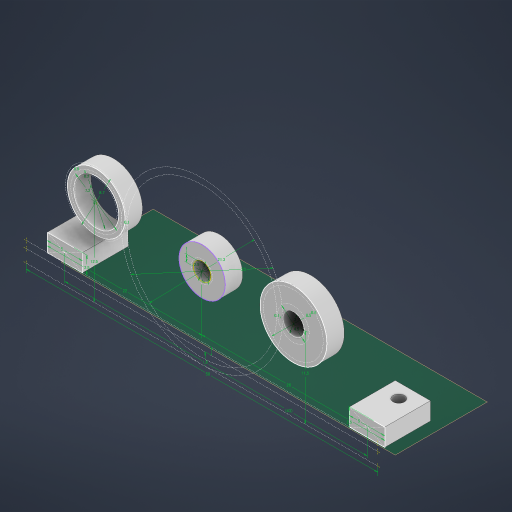
# Autodesk Inventor part: motormount
Saved by Autodesk Inventor 2023.5 (Build 275446000, 446)
## iProperties
Created: 2025-01-19
Part Number: motormount
Material: 一般
Document SubType Name: Modeling
Designer: IshiiLabHonda
Density: 1 g/cm^3
Appearance: 既定
Author: IshiiLabHonda
Autodesk Inventor part; units mm, degrees
ref_plane "YZ Plane" through (0, 0, 0) normal (1, 0, 0) x (0, 1, 0)
ref_plane "XZ Plane" through (0, 0, 0) normal (0, 1, 0) x (-1, 0, 0)
ref_plane "XY Plane" through (0, 0, 0) normal (0, 0, 1) x (1, 0, 0)
sketch "スケッチ1" plane through (0, 0, 0) normal (0, 0, 1) x (1, 0, 0)
  circle A0 centre (0, 0) radius 10.65 construction
  line L0 (0, 0) -> (0, 1) construction
  line L1 (0, 0) -> (1, 0) construction
  circle A1 centre (13, 0) radius 2.25 construction
  circle A2 centre (-15.0669, 1) radius 4.35 construction
  circle A3 centre (0, 0) radius 11.5 construction
  line L2 (-25, -11.5) -> (25, -11.5) construction
  line L3 (-25, -9.7) -> (25, -9.7) construction
  line L4 (-25, -8.7) -> (25, -8.7) construction
  dimension "d0" = 1
  dimension "d2" = 1
  dimension "d3" = 21.3
  dimension "d5" = 4.5
  dimension "d6" = 0.1
  dimension "d7" = 8.7
  dimension "d8" = 0.1
  dimension "d9" = 23
  dimension "d10" = 50
  dimension "d11" = 1.8
  dimension "d12" = 1
  dimension "d46" = 12.5
  dimension "d47" = 11.5
  constraints: 10 end point, 5 parallel, 4 centre point, 4 coincident, 3 symmetric about line, 1 perpendicular, 1 tangent, 1 vertical
  measures "d0" distance of L0.start L0.end
  measures "d2" distance of L0.start L1.end
  measures "d3" diameter of A0
  measures "d5" diameter of A1
  measures "d7" diameter of A2
  measures "d9" diameter of A3
  measures "d10" distance of L2.start L2.end
  measures "d11" distance between parallel lines of L2 L3
  measures "d12" distance between parallel lines of L3 L4
  measures "d46" distance from line of L2 A2.centre
  measures "d47" distance from line of L2 A1.centre
sketch "スケッチ2" plane through (0, 0, 0) normal (0, 0, 1) x (1, 0, 0)
  circle A0 centre (-15.0669, 1) radius 4.35 construction
  line L0 (0, 0) -> (0, 1) construction
  circle A1 centre (0, 0) radius 10.65 construction
  circle A2 centre (0, 0) radius 11.5 construction
  line L1 (-25, -8.7) -> (25, -8.7) construction
  line L2 (-25, -9.7) -> (25, -9.7) construction
  line L3 (-25, -11.5) -> (25, -11.5) construction
  line L4 (0, 0) -> (1, 0) construction
  circle A3 centre (13, 0) radius 2.25 construction
  circle A4 centre (13, 0) radius 4.25 construction
  circle A5 centre (-15.0669, 1) radius 3.6 construction
  circle A6 centre (-15.0669, 1) radius 3 construction
  circle A7 centre (0, 0) radius 1.25 construction
  circle A8 centre (0, 0) radius 1.5 construction
  dimension "d13" = 8.5
  dimension "d14" = 7.2
  dimension "d15" = 6
  dimension "d27" = 2.5
  dimension "d28" = 3
  constraints: 5 centre point, 5 coincident
  measures "d13" diameter of A4
  measures "d14" diameter of A5
  measures "d15" diameter of A6
  measures "d27" diameter of A7
  measures "d28" diameter of A8
sketch "スケッチ3" plane through (0, 0, 0) normal (0, 0, 1) x (1, 0, 0)
  circle A0 centre (-15.0669, 1) radius 4.35 construction
  line L0 (0, 0) -> (0, 1) construction
  line L1 (0, 0) -> (1, 0) construction
  line L2 (-25, -11.5) -> (25, -11.5) construction
  line L3 (-25, -9.7) -> (25, -9.7) construction
  line L4 (-25, -8.7) -> (25, -8.7) construction
  circle A1 centre (13, 0) radius 2.25 construction
  circle A2 centre (0, 0) radius 10.65 construction
  circle A3 centre (0, 0) radius 11.5 construction
  circle A4 centre (-15.0669, 1) radius 4.35 construction
  line L5 (0, 0) -> (0, 1) construction
  circle A5 centre (0, 0) radius 10.65 construction
  circle A6 centre (0, 0) radius 11.5 construction
  line L6 (-25, -8.7) -> (25, -8.7) construction
  line L7 (-25, -9.7) -> (25, -9.7) construction
  line L8 (-25, -11.5) -> (25, -11.5) construction
  line L9 (0, 0) -> (1, 0) construction
  circle A7 centre (13, 0) radius 2.25 construction
  circle A8 centre (13, 0) radius 4.25 construction
  circle A9 centre (-15.0669, 1) radius 3.6 construction
  circle A10 centre (-15.0669, 1) radius 3 construction
  line L10 (-22, -6.2) -> (-17, -6.2)
  line L11 (-17, -6.2) -> (-17, -8.7)
  line L12 (-22, -8.7) -> (-22, -6.2)
  line L13 (21, -6.2) -> (26, -6.2)
  line L14 (26, -6.2) -> (26, -8.7)
  line L15 (21, -8.7) -> (21, -6.2)
  line L16 (-22, -6.2) -> (-17, -8.7) construction
  line L17 (-22, -8.7) -> (-17, -6.2) construction
  line L18 (21, -6.2) -> (26, -8.7) construction
  line L19 (21, -8.7) -> (26, -6.2) construction
  line L20 (-22, -8.7) -> (-17, -8.7)
  line L21 (21, -8.7) -> (26, -8.7)
  circle A11 centre (-15.0669, 1) radius 3.2
  circle A12 centre (-15.0669, 1) radius 4.1
  circle A13 centre (13, 0) radius 4.75
  circle A14 centre (0, 0) radius 3.2895
  circle A15 centre (0, 0) radius 1.25 projected
  circle A16 centre (13, 0) radius 1.5
  point P0 (-19.5, -7.45)
  point P1 (23.5, -7.45)
  point P2 (15.3415, -6)
  point P3 (15, -6.1912)
  dimension "d17" = 5
  dimension "d18" = 5
  dimension "d19" = 2.5
  dimension "d20" = 2.5
  dimension "d22" = 22
  dimension "d23" = 26
  dimension "d24" = 0.2
  dimension "d25" = 0.5
  dimension "d26" = 0.5
  dimension "d31" = 3
  dimension "d39" = 43
  constraints: 24 end point, 5 centre point, 5 coincident, 4 point on line, 3 parallel, 2 midpoint, 2 perpendicular, 4 other
  measures "d17" distance between parallel lines of L11 L12
  measures "d18" distance between parallel lines of L15 L14
  measures "d19" distance between parallel lines of L6 L10
  measures "d20" distance between parallel lines of L4 L13
  measures "d22" distance of the line from the sketch origin of L12
  measures "d23" distance of the line from the sketch origin of L14
  measures "d24" radial gap between concentric circles of A10 A11
  measures "d25" radial gap between concentric circles of A12 A9
  measures "d26" radial gap between concentric circles of A8 A13
  measures "d31" diameter of A16
  measures "d39" distance of point (23.5, -7.45) point (-19.5, -7.45)
extrude "押し出し1" add sketch "スケッチ3" against normal blind 6.5 contours L10 L11 L20 L12 | L13 L14 L21 L15
extrude "押し出し2" add sketch "スケッチ3" against normal blind 2.5 contours A12 | A13 | A14
ref_plane "作業平面1" through (21, -8.7, 0) normal (0, -1, 0) x (1, 0, 0)
sketch "スケッチ4" plane through (21, -8.7, 0) normal (0, -1, 0) x (1, 0, 0)
  line L0 (0, 0) -> (5, 0) projected
  line L1 (0, 0) -> (0, -6.5) projected
  line L2 (5, -6.5) -> (0, -6.5) projected
  line L3 (5, 0) -> (5, -6.5) projected
  line L4 (-43, 0) -> (-38, 0) projected
  line L5 (-43, 0) -> (-43, -6.5) projected
  line L6 (-38, -6.5) -> (-43, -6.5) projected
  line L7 (-38, 0) -> (-38, -6.5) projected
  line L8 (5, 0) -> (0, 0) projected
  line L9 (0, 0) -> (0, -6.5) projected
  line L10 (5, 0) -> (5, -6.5) projected
  line L11 (-43, 0) -> (-38, 0) projected
  circle A0 centre (2.5, -4.5) radius 0.8
  circle A1 centre (-40.5, -4.5) radius 0.8
  line L12 (-43, 0) -> (-43, -6.5) projected
  line L13 (-43, -2.5) -> (-38, -2.5)
  line L14 (0, -2.5) -> (5, -2.5)
  line L15 (-43, -2.5) -> (-38, -6.5) construction
  line L16 (-38, -6.5) -> (-43, -6.5) projected
  line L17 (-43, -6.5) -> (-38, -2.5) construction
  line L18 (0, -6.5) -> (5, -6.5) projected
  line L19 (0, -2.5) -> (5, -6.5) construction
  line L20 (0, -6.5) -> (5, -2.5) construction
  point P0 (-21, 0)
  dimension "d35" = 1.6
  dimension "d36" = 1.6
  dimension "d44" = 2.5
  dimension "d45" = 2.5
  constraints: 12 end point, 4 point on line, 2 centre point, 2 coincident, 2 midpoint, 2 perpendicular
  measures "d35" diameter of A0
  measures "d36" diameter of A1
  measures "d44" distance between parallel lines of L0 L14
  measures "d45" distance between parallel lines of L4 L13
extrude "押し出し3" cut sketch "スケッチ4" against normal up to surface (2.5 mm away) contours A0 | A1
equation "\"d2\" = d0"
equation "\"d36\" = d35"
